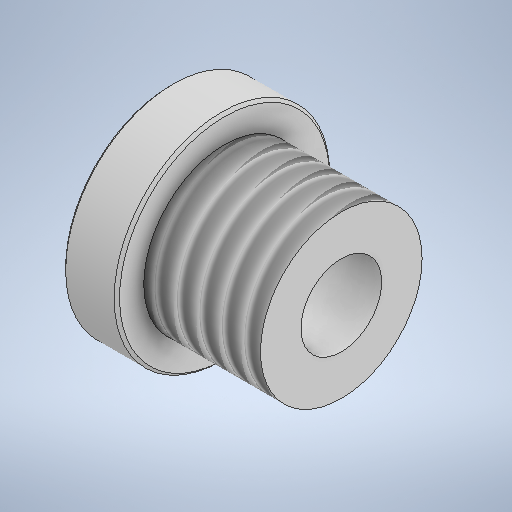
# Autodesk Inventor part: 1102
Saved by Autodesk Inventor 2025.1 (Build 291241000, 241)
## iProperties
Created: 2024-06-07
Part Number: 1102
Material: Generisch
Document SubType Name: Modeling
Designer: ffogue
Density: 1 g/cm^3
Appearance: Vorgabe
Author: ffogue
Autodesk Inventor part; units mm, degrees
ref_plane "YZ Plane" through (0, 0, 0) normal (1, 0, 0) x (0, 1, 0)
ref_plane "XZ Plane" through (0, 0, 0) normal (0, 1, 0) x (-1, 0, 0)
sketch "Skizze1" plane through (0, 0, 0) normal (0, 1, 0) x (-1, 0, 0)
  line L0 (0, 0) -> (0, 12)
  line L1 (0, 12) -> (-6, 12)
  line L2 (-6, 12) -> (-6, 9)
  line L3 (-6, 9) -> (-19, 9)
  line L4 (-19, 9) -> (-19, 0)
  line L5 (-19, 0) -> (0, 0)
  dimension "d0" = 24
  dimension "d1" = 18
  dimension "d2" = 6
  dimension "d3" = 13
  constraints: 12 end point, 5 perpendicular, 1 vertical
  measures "d0" diameter of L1 L5
  measures "d1" diameter of L3 L5
  measures "d2" distance between parallel lines of L0 L2
  measures "d3" distance between parallel lines of L4 L2
revolve "Umdrehung1" add sketch "Skizze1" angle 360 about axis through (19, 0, 0) along (-1, 0, 0)
sketch "Skizze2" plane through (19, 0, 0) normal (1, 0, 0) x (0, 0, -1)
  circle A0 centre (0, 0) radius 9 projected
  constraints: 1 coincident
hole "Bohrung1" at (19, 0, 0) direction (-1, 0, 0) diameter 9 depth 19
thread "Gewinde1" size "M18x2.5" class "6g" standard "ISO Metric profile" length 18
ref_plane "Arbeitsebene1" through (0, 0, 12) normal (0, 0, 1) x (1, 0, 0)
chamfer "Fasen1" distance 0.3 angle 45 2 edges at (0, 0, -12) (6, 0, -12)
